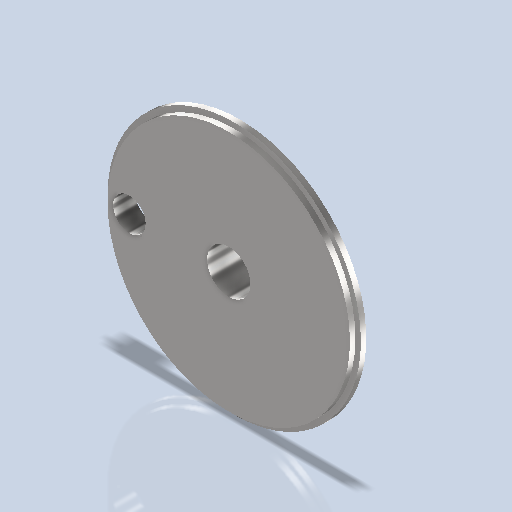
# Autodesk Inventor part: 5
Saved by Autodesk Inventor 2024.2 (Build 282272000, 272)
## iProperties
Created: 2024-05-04
Part Number: 5
Material: Stahl, Kohlenstoff
Document SubType Name: Modeling
Designer: Fabri
Density: 7.85 g/cm^3
Appearance: Halbpoliert
Author: Fabri
Autodesk Inventor part; units mm, degrees
ref_plane "YZ Plane" through (0, 0, 0) normal (1, 0, 0) x (0, 1, 0)
ref_plane "XZ Plane" through (0, 0, 0) normal (0, 1, 0) x (-1, 0, 0)
ref_plane "XY Plane" through (0, 0, 0) normal (0, 0, 1) x (1, 0, 0)
sketch "Skizze1" plane through (0, 0, 0) normal (0, 1, 0) x (-1, 0, 0)
  circle A0 centre (0, 0) radius 116.25
  circle A1 centre (0, 0) radius 111.25
  dimension "d0" = 222.5
  dimension "d1" = 232.5
  constraints: 2 centre point, 2 coincident
  measures "d0" diameter of A1
  measures "d1" diameter of A0
extrude "Extrusion1" add sketch "Skizze1" against normal blind 5 contours A1
extrude "Extrusion2" add sketch "Skizze1" along normal blind 5 contours A0 | A1
sketch "Skizze2" plane through (0, 5, 0) normal (0, 1, 0) x (1, 0, 0)
  circle A0 centre (0, 0) radius 111.25 projected
  circle A1 centre (0, 0) radius 25
  circle A2 centre (0, 0) radius 20
  dimension "d6" = 50
  dimension "d7" = 40
  constraints: 2 centre point, 2 coincident
  measures "d6" diameter of A1
  measures "d7" diameter of A2
extrude "Extrusion3" add sketch "Skizze2" along normal blind 20 contours A1
sketch "Skizze3" plane through (0, -5, 0) normal (0, -1, 0) x (1, 0, 0)
  circle A0 centre (-91.25, 0) radius 20
  circle A1 centre (-91.25, 0) radius 15
  circle A2 centre (0, 0) radius 111.25 projected
  dimension "d14" = 40
  dimension "d15" = 30
  constraints: 2 centre point, 1 coincident, 1 horizontal alignment, 1 tangent
  measures "d14" diameter of A0
  measures "d15" diameter of A1
extrude "Extrusion5" add sketch "Skizze3" against normal blind 20 contours A0
sketch "Skizze4" plane through (-91.25, 5, 0) normal (0, 1, 0) x (1, 0, 0)
  circle A0 centre (0, 0) radius 15 projected
  circle A1 centre (91.25, 0) radius 20 projected
extrude "Extrusion6" cut sketch "Skizze4" against normal up to surface (10 mm away)
sketch "Skizze5" plane through (0, 25, 0) normal (0, 1, 0) x (1, 0, 0)
  circle A0 centre (0, 0) radius 20 projected
extrude "Extrusion7" add sketch "Skizze5" along normal blind 20
fillet "Rundung1" radius 5 1 edges at (-20, 45, 0)
